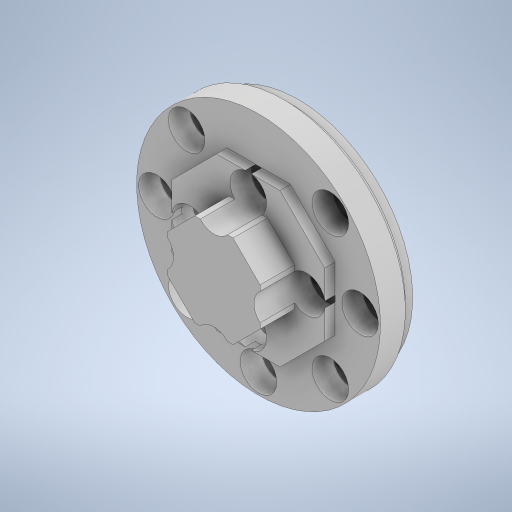
# Autodesk Inventor part: acc_motor_drive_mount
Saved by Autodesk Inventor 2023.4 (Build 274418000, 418)
## iProperties
Created: 2023-11-23
Part Number: acc_motor_drive_mount
Material: Generic
Document SubType Name: Modeling
Designer: aaron
Density: 1 g/cm^3
Appearance: Default
Author: aaron
Autodesk Inventor part; units mm, degrees
ref_plane "YZ Plane" through (0, 0, 0) normal (1, 0, 0) x (0, 1, 0)
ref_plane "XZ Plane" through (0, 0, 0) normal (0, 1, 0) x (-1, 0, 0)
ref_plane "XY Plane" through (0, 0, 0) normal (0, 0, 1) x (1, 0, 0)
sketch "Sketch1" plane through (0, 0, 0) normal (0, 0, 1) x (1, 0, 0)
  circle A0 centre (0, 0) radius 22.55
  dimension "d0" = 45.1
  constraints: 1 centre point, 1 coincident
  measures "d0" diameter of A0
extrude "Extrusion1" add sketch "Sketch1" along normal blind 3
sketch "Sketch2" plane through (0, 0, 3) normal (0, 0, 1) x (1, 0, 0)
  circle A0 centre (0, 0) radius 14.5
  dimension "d3" = 29
  constraints: 1 centre point, 1 coincident
  measures "d3" diameter of A0
extrude "Extrusion2" cut sketch "Sketch2" against normal through all
chamfer "Chamfer1" distance 0.5 angle 45 3 edges at (-14.5, 0, 3) (-14.5, 0, 0) (-22.55, 0, 0)
sketch "Sketch3" plane through (0, 0, 3) normal (0, 0, 1) x (1, 0, 0)
  circle A0 centre (-14.1421, 14.1421) radius 2
  circle A1 centre (14.1421, 14.1421) radius 2
  circle A2 centre (20, 0) radius 2
  circle A3 centre (14.1421, -14.1421) radius 2
  circle A4 centre (0, -20) radius 2
  circle A5 centre (-14.1421, -14.1421) radius 2
  circle A6 centre (-20, 0) radius 2
  line L0 (-9.1, -3.7693) -> (-9.1, 3.7693)
  line L1 (-9.1, 3.7693) -> (-3.7693, 9.1)
  line L2 (-3.7693, 9.1) -> (3.7693, 9.1)
  line L3 (3.7693, 9.1) -> (9.1, 3.7693)
  line L4 (9.1, 3.7693) -> (9.1, -3.7693)
  line L5 (9.1, -3.7693) -> (3.7693, -9.1)
  line L6 (3.7693, -9.1) -> (-3.7693, -9.1)
  line L7 (-3.7693, -9.1) -> (-9.1, -3.7693)
  line L8 (3.7486, 9.05) -> (-3.7486, 9.05)
  line L9 (-3.7486, 9.05) -> (-9.05, 3.7486)
  line L10 (-9.05, 3.7486) -> (-9.05, -3.7486)
  line L11 (-9.05, -3.7486) -> (-3.7486, -9.05)
  line L12 (-3.7486, -9.05) -> (3.7486, -9.05)
  line L13 (3.7486, -9.05) -> (9.05, -3.7486)
  line L14 (9.05, -3.7486) -> (9.05, 3.7486)
  line L15 (9.05, 3.7486) -> (3.7486, 9.05)
  circle A7 centre (0, 0) radius 24
  dimension "d9" = 0.05
  dimension "d21" = 48
  dimension "d22" = 4
  dimension "d23" = 4
  dimension "d24" = 4
  dimension "d25" = 4
  dimension "d26" = 4
  dimension "d27" = 4
  dimension "d28" = 4
  constraints: 32 end point, 8 centre point, 1 coincident, 7 other
  measures "d9" distance between parallel lines of L2 L8
  measures "d21" diameter of A7
  measures "d22" diameter of A5
  measures "d23" diameter of A4
  measures "d24" diameter of A3
  measures "d25" diameter of A2
  measures "d26" diameter of A1
  measures "d27" diameter of A0
  measures "d28" diameter of A6
extrude "Extrusion3" add sketch "Sketch3" along normal blind 7.8 contours A7
sketch "Sketch4" plane through (0, 0, 10.8) normal (0, 0, 1) x (1, 0, 0)
  line L0 (-9.1, 3.7693) -> (-3.7693, 9.1) projected
  line L1 (-3.7693, 9.1) -> (3.7693, 9.1) projected
  line L2 (3.7693, 9.1) -> (9.1, 3.7693) projected
  line L3 (9.1, 3.7693) -> (9.1, -3.7693) projected
  line L4 (9.1, -3.7693) -> (3.7693, -9.1) projected
  line L5 (3.7693, -9.1) -> (-3.7693, -9.1) projected
  line L6 (-3.7693, -9.1) -> (-9.1, -3.7693) projected
  line L7 (-9.1, -3.7693) -> (-9.1, 3.7693) projected
  point P0 (0, 0)
extrude "Extrusion4" add sketch "Sketch4" along normal mid plane 12
sketch "Sketch5" plane through (0, 0, 16.8) normal (0, 0, 1) x (1, 0, 0)
  line L0 (-9.1, -3.7693) -> (-3.7693, -9.1) projected
  line L1 (-3.7693, -9.1) -> (3.7693, -9.1) projected
  line L2 (3.7693, -9.1) -> (9.1, -3.7693) projected
  line L3 (9.1, -3.7693) -> (9.1, 3.7693) projected
  line L4 (9.1, 3.7693) -> (3.7693, 9.1) projected
  line L5 (3.7693, 9.1) -> (-3.7693, 9.1) projected
  line L6 (-3.7693, 9.1) -> (-9.1, 3.7693) projected
  line L7 (-9.1, 3.7693) -> (-9.1, -3.7693) projected
  point P0 (0, 0)
extrude "Extrusion5" add sketch "Sketch5" along normal blind 2.8
sketch "Sketch6" plane through (0, 0, 10.8) normal (0, 0, 1) x (1, 0, 0)
  line L0 (-15.1, 6.2546) -> (-6.2546, 15.1)
  line L1 (-15.1, -6.2546) -> (-15.1, 6.2546)
  line L2 (-6.2546, -15.1) -> (-15.1, -6.2546)
  line L3 (6.2546, -15.1) -> (-6.2546, -15.1)
  line L4 (15.1, -6.2546) -> (6.2546, -15.1)
  line L5 (15.1, 6.2546) -> (15.1, -6.2546)
  line L6 (6.2546, 15.1) -> (15.1, 6.2546)
  line L7 (-6.2546, 15.1) -> (6.2546, 15.1)
  line L8 (6.2339, 15.05) -> (15.05, 6.2339)
  line L9 (15.05, 6.2339) -> (15.05, -6.2339)
  line L10 (15.05, -6.2339) -> (6.2339, -15.05)
  line L11 (6.2339, -15.05) -> (-6.2339, -15.05)
  line L12 (-6.2339, -15.05) -> (-15.05, -6.2339)
  line L13 (-15.05, -6.2339) -> (-15.05, 6.2339)
  line L14 (-15.05, 6.2339) -> (-6.2339, 15.05)
  line L15 (-6.2339, 15.05) -> (6.2339, 15.05)
  point P0 (0, 0)
  point P1 (0, 0)
  point P2 (0, 0)
  dimension "d16" = 0.05
  constraints: 32 end point, 7 other
  measures "d16" distance between parallel lines of L7 L15
extrude "Extrusion6" add sketch "Sketch6" along normal blind 2 contours L8 L9 L10 L11 L12 L13 L14 L15
sketch "Sketch7" plane through (0, 0, 0) normal (0, 0, -1) x (-1, 0, 0)
  circle A0 centre (0, 0) radius 22.55 projected
  circle A1 centre (0, 0) radius 24 projected
extrude "Extrusion7" cut sketch "Sketch7" against normal blind 4.8
sketch "Sketch8" plane through (0, 0, 0) normal (0, 0, -1) x (-1, 0, 0)
  circle A0 centre (0, 0) radius 5.45
  dimension "d29" = 10.9
  constraints: 1 centre point, 1 coincident
  measures "d29" diameter of A0
extrude "Extrusion8" add sketch "Sketch8" against normal up to surface (3 mm away)
chamfer "Chamfer2" distance 1.1 angle 45 1 edges at (-24, 0, 4.8)
chamfer "Chamfer3" distance 0.2 angle 45 1 edges at (22.55, 0, 4.8)
sketch "Sketch9" plane through (0, 0, 19.6) normal (0, 0, 1) x (1, 0, 0)
  circle A0 centre (0, 0) radius 11.5
  line L0 (0, 0) -> (0, -13.9959)
  circle A1 centre (0, -11.5) radius 2
  circle A2 centre (11.5, 0) radius 2
  circle A3 centre (0, 11.5) radius 2
  circle A4 centre (-11.5, 0) radius 2
  dimension "d38" = 23
  dimension "d39" = 4
  dimension "d42" = 360
  constraints: 4 centre point, 2 end point, 1 coincident, 1 point on line, 1 vertical, 1 vertical alignment, 11 other
  measures "d39" diameter of A1
extrude "Extrusion9" cut sketch "Sketch9" against normal through all contours A0 A2 | A0 A2 | A3 A0 | A0 A3 | A1 L0 A0 | A0 L0 A1 | L0 A1 A0 | A0 A1 L0 | A4 A0 | A0 A4
sketch "Sketch10" plane through (0, 0, 12.8) normal (0, 0, 1) x (1, 0, 0)
  circle A0 centre (0, -11.5) radius 2 projected
  circle A1 centre (0, -11.5) radius 3.6
  circle A2 centre (11.5, 0) radius 3.6
  circle A3 centre (0, 11.5) radius 3.6
  circle A4 centre (-11.5, 0) radius 3.6
  point P0 (0, 0)
  dimension "d46" = 7.2
  dimension "d49" = 360
  constraints: 4 centre point, 1 coincident, 9 other
  measures "d46" diameter of A1
extrude "Extrusion10" cut sketch "Sketch10" along normal mid plane 8.4
sketch "Sketch12" plane through (0, 0, 10.8) normal (0, 0, 1) x (1, 0, 0)
  circle A0 centre (-14.1421, 14.1421) radius 2 projected
  circle A1 centre (-14.1421, 14.1421) radius 3.6
  circle A2 centre (-20, 0) radius 3.6
  circle A3 centre (-14.1421, -14.1421) radius 3.6
  circle A4 centre (0, -20) radius 3.6
  circle A5 centre (14.1421, -14.1421) radius 3.6
  circle A6 centre (20, 0) radius 3.6
  circle A7 centre (14.1421, 14.1421) radius 3.6
  circle A8 centre (0, 20) radius 3.6
  point P0 (0, 0)
  dimension "d53" = 7.2
  dimension "d56" = 360
  constraints: 8 centre point, 1 coincident, 17 other
  measures "d53" diameter of A1
extrude "Extrusion11" cut sketch "Sketch12" against normal blind 4.2 contours A1 | A2 | A3 | A4 | A5 | A6 | A7
sketch "Sketch14" plane through (0, 0, 19.6) normal (0, 0, 1) x (1, 0, 0)
  arc A0 (-2.6833, 9.1) -> (2.6833, 9.1) centre (0, 11.5) ccw projected
  line L0 (3.7693, 9.1) -> (-3.7693, 9.1) projected
  arc A1 (9.1, 2.6833) -> (9.1, -2.6833) centre (11.5, 0) ccw projected
  line L1 (9.1, -3.7693) -> (9.1, 3.7693) projected
  arc A2 (2.6833, -9.1) -> (-2.6833, -9.1) centre (0, -11.5) ccw projected
  line L2 (-3.7693, -9.1) -> (3.7693, -9.1) projected
  arc A3 (-9.1, -2.6833) -> (-9.1, 2.6833) centre (-11.5, 0) ccw projected
  line L3 (-9.1, 3.7693) -> (-9.1, -3.7693) projected
  point P0 (0, 0)
extrude "Extrusion12" cut sketch "Sketch14" against normal up to surface (11 mm away)
sketch "Sketch15" plane through (0, 0, 0) normal (0, 0, -1) x (-1, 0, 0)
  circle A0 centre (0, 0) radius 38.822
  constraints: 1 centre point, 1 coincident
extrude "Extrusion13" cut sketch "Sketch15" against normal up to surface (3 mm away)
equation "\"d23\" = d22"
equation "\"d24\" = d22"
equation "\"d25\" = d22"
equation "\"d26\" = d22"
equation "\"d27\" = d22"
equation "\"d28\" = d22"
body "Solid1"
